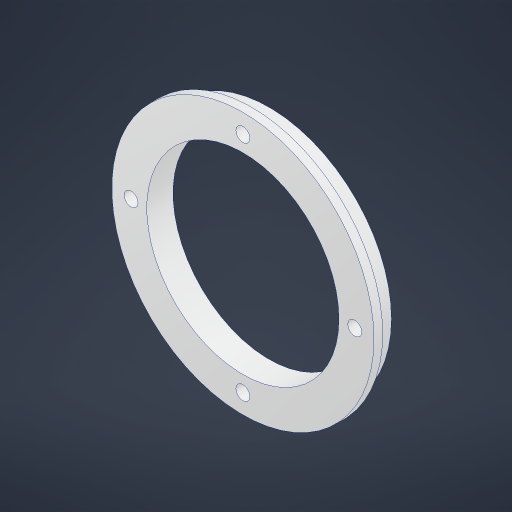
# Autodesk Inventor part: LS-002
Saved by Autodesk Inventor 2023.4 (Build 274418000, 418)
## iProperties
Created: 2025-03-08
Part Number: LS-002
Material: Aluminum 6061
Document SubType Name: Modeling
Designer: jmcintyr
Density: 2.7 g/cm^3
Appearance: Aluminum - Flat
Author: jmcintyr
Autodesk Inventor part; units mm, degrees
ref_plane "YZ Plane" through (0, 0, 0) normal (1, 0, 0) x (0, 1, 0)
ref_plane "XZ Plane" through (0, 0, 0) normal (0, 1, 0) x (-1, 0, 0)
ref_plane "XY Plane" through (0, 0, 0) normal (0, 0, 1) x (1, 0, 0)
sketch "Sketch1" plane through (0, 0, 0) normal (0, 0, 1) x (1, 0, 0)
  circle A0 centre (0, 0) radius 44.45
  circle A1 centre (0, 0) radius 34.925
  dimension "d0" = 88.9
  dimension "d20" = 69.85
  constraints: 2 centre point, 1 coincident
  measures "d0" diameter of A0
  measures "d20" diameter of A1
extrude "Extrusion1" add sketch "Sketch1" against normal blind 6.35
sketch "Sketch3" plane through (0, 0, 0) normal (0, 0, 1) x (1, 0, 0)
  circle A0 centre (0, 0) radius 41.402 construction
  line L0 (0, 0) -> (29.2756, 29.2756) construction
  circle A1 centre (0, 0) radius 44.45 construction
  line L1 (-44.45, 0) -> (44.45, 0) construction
  point P0 (-29.2756, 29.2756)
  point P1 (-29.2756, -29.2756)
  point P2 (29.2756, -29.2756)
  dimension "d4" = 82.804
  dimension "d5" = 45
  dimension "d8" = 360
  constraints: 4 end point, 2 point on circle, 1 coincident, 1 horizontal, 8 other
  measures "d5" angle of L1 L0
hole "Hole1" at (29.2756, 29.2756, 0) at (-29.2756, 29.2756, 0) at (-29.2756, -29.2756, 0) at (29.2756, -29.2756, 0) direction (0, 0, -1) diameter 3.9624 end through all thread size "10-32 UNF" class "2B" standard "ANSI Unified Screw Threads"
sketch "Sketch7" plane through (0, 0, 0) normal (0, 0, 1) x (1, 0, 0)
  circle A0 centre (0, 0) radius 34.925 projected
  circle A1 centre (0, 0) radius 47.625
  dimension "d25" = 95.25
  constraints: 1 centre point, 1 coincident
  measures "d25" diameter of A1
extrude "Extrusion4" add sketch "Sketch7" along normal blind 3.175
sketch "Sketch8" plane through (0, 0, 3.175) normal (0, 0, 1) x (1, 0, 0)
  circle A0 centre (0, 0) radius 40.64 construction
  point P0 (40.64, 0)
  point P1 (0, 40.64)
  point P2 (-40.64, 0)
  point P3 (0, -40.64)
  dimension "d28" = 81.28
  dimension "d38" = 360
  constraints: 2 coincident, 1 horizontal alignment, 7 other
hole "Hole2" at (0, 40.64, 3.175) at (-40.64, 0, 3.175) at (0, -40.64, 3.175) at (40.64, 0, 3.175) direction (0, 0, -1) diameter 5.1054 end through all
body "Solid1"
